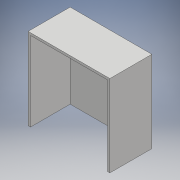
# Autodesk Inventor part: こたつ
Saved by Autodesk Inventor 2018 (Build 220112000, 112)
## iProperties
Created: 2017-10-19
Part Number: こたつ
Material: 一般
Document SubType Name: Modeling
Designer: mura5
Density: 1 g/cm^3
Appearance: 既定
Author: mura5
Autodesk Inventor part; units mm, degrees
ref_plane "YZ Plane" through (0, 0, 0) normal (1, 0, 0) x (0, 1, 0)
ref_plane "XZ Plane" through (0, 0, 0) normal (0, 1, 0) x (-1, 0, 0)
ref_plane "XY Plane" through (0, 0, 0) normal (0, 0, 1) x (1, 0, 0)
sketch "スケッチ1" plane through (0, 0, 0) normal (0, 1, 0) x (-1, 0, 0)
  line L0 (-350, 350) -> (350, 350)
  line L1 (350, 350) -> (350, -350)
  line L2 (350, -350) -> (-350, -350)
  line L3 (-350, -350) -> (-350, 350)
  line L4 (-350, 350) -> (350, -350) construction
  line L5 (350, 350) -> (-350, -350) construction
  point P0 (0, 0)
  dimension "d0" = 700
  dimension "d1" = 700
  constraints: 12 end point, 2 midpoint, 2 parallel, 1 horizontal, 1 perpendicular
  measures "d0" distance of L1.end L2.end
  measures "d1" distance of L0.end L1.end
extrude "押し出し1" add sketch "スケッチ1" along normal blind 20
sketch "スケッチ2" plane through (350, 0, 350) normal (1, 0, 0) x (0, 0, -1)
  line L0 (0, 0) -> (0, 20) projected
  line L1 (0, 0) -> (700, 0)
  line L2 (700, 0) -> (700, -340)
  line L3 (700, -340) -> (0, -340)
  line L4 (0, -340) -> (0, 0)
  point P0 (350, 0)
  dimension "d4" = 700
  dimension "d5" = 340
  constraints: 8 end point, 2 parallel, 1 horizontal, 1 perpendicular
  measures "d4" distance of L2.end L3.end
  measures "d5" distance of L1.end L2.end
extrude "押し出し2" add sketch "スケッチ2" against normal blind 20
sketch "スケッチ3" plane through (-350, 0, -350) normal (-1, 0, 0) x (0, 0, 1)
  line L0 (0, 20) -> (0, -340) projected
  line L1 (0, -340) -> (700, -340) projected
  line L2 (0, 0) -> (700, 0)
  line L3 (700, 0) -> (700, -340)
  line L4 (700, -340) -> (0, -340)
  line L5 (0, -340) -> (0, 0)
  point P0 (350, 0)
  constraints: 8 end point, 2 parallel, 1 horizontal, 1 perpendicular, 1 point on line
extrude "押し出し3" add sketch "スケッチ3" against normal blind 20
sketch "スケッチ4" plane through (-350, 20, 350) normal (0, 0, 1) x (1, 0, 0)
  line L0 (20, -20) -> (20, -360) projected
  line L1 (680, -360) -> (680, -20) projected
  line L2 (20, -20) -> (680, -20)
  line L3 (680, -20) -> (680, -360)
  line L4 (680, -360) -> (20, -360)
  line L5 (20, -360) -> (20, -20)
  point P0 (350, -20)
  constraints: 8 end point, 2 parallel, 1 horizontal, 1 perpendicular
extrude "押し出し4" add sketch "スケッチ4" against normal blind 20
